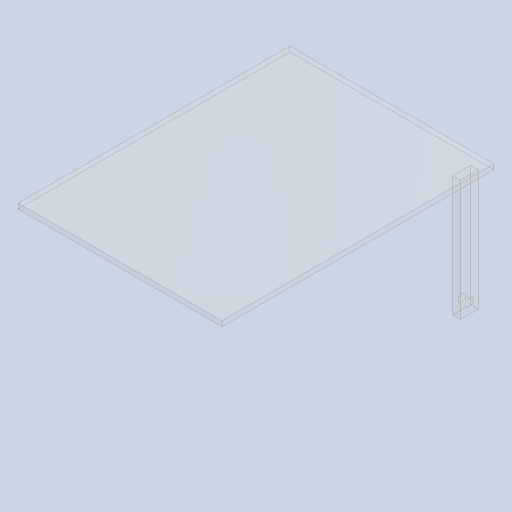
# Autodesk Inventor part: Enclosure Lid
Saved by Autodesk Inventor 2024 (Build 280153000, 153)
## iProperties
Created: 2025-03-05
Part Number: Enclosure Lid
Material: Generic
Document SubType Name: Modeling
Designer: Kemper Room 121
Density: 1 g/cm^3
Appearance: Polycarbonate - Clear
Author: Kemper Room 121
Autodesk Inventor part; units mm, degrees
ref_plane "YZ Plane" through (0, 0, 0) normal (1, 0, 0) x (0, 1, 0)
ref_plane "XZ Plane" through (0, 0, 0) normal (0, 1, 0) x (-1, 0, 0)
ref_plane "XY Plane" through (0, 0, 0) normal (0, 0, 1) x (1, 0, 0)
sketch "Sketch1" plane through (0, 0, 0) normal (0, 1, 0) x (-1, 0, 0)
  line L0 (0, 0) -> (79.5, 0)
  line L1 (79.5, 0) -> (79.5, -106)
  line L2 (79.5, -106) -> (0, -106)
  line L3 (0, -106) -> (0, 0)
  dimension "d6" = 106
  dimension "d7" = 79.5
  constraints: 8 end point, 2 parallel, 1 horizontal, 1 perpendicular
  measures "d6" distance of L0.end L1.end
  measures "d7" distance of L0.start L0.end
extrude "Extrusion1" add sketch "Sketch1" along normal blind 2
sketch "Sketch2" plane through (0, 0, 0) normal (0, -1, 0) x (1, 0, 0)
  line L0 (0, -106) -> (-79.5, -106) projected
  line L1 (0, 0) -> (0, -106) projected
  line L2 (-79.5, 0) -> (0, 0) projected
  line L3 (-79.5, -106) -> (-79.5, 0) projected
  line L4 (-3, -103) -> (-6, -103)
  line L5 (-6, -103) -> (-6, -96)
  line L6 (-6, -96) -> (-3, -96)
  line L7 (-3, -96) -> (-3, -103)
  dimension "d10" = 7
  dimension "d11" = 3
  dimension "d12" = 3
  dimension "d13" = 3
  constraints: 8 end point, 2 parallel, 1 horizontal, 1 perpendicular
  measures "d10" distance of L6.end L4.start
  measures "d11" distance between parallel lines of L1 L7
  measures "d12" distance between parallel lines of L0 L4
  measures "d13" distance of L4.start L4.end
extrude "Extrusion2" add sketch "Sketch2" along normal blind 48 contours L4 L5 L6 L7
sketch "Sketch3" plane through (-3, 0, -96) normal (1, 0, 0) x (0, 0, -1)
  circle A0 centre (3.5, -43) radius 1.5
  line L0 (7, -48) -> (0, -48) projected
  line L1 (7, 0) -> (7, -48) projected
  point P0 (-96, 0)
  dimension "d14" = 5
  dimension "d16" = 3
  dimension "d22" = 3.5
  constraints: 1 centre point
  measures "d14" distance from line of L0 A0.centre
  measures "d16" diameter of A0
  measures "d22" distance from line of L1 A0.centre
extrude "Extrusion3" cut sketch "Sketch3" against normal blind 33
sketch "Sketch4" plane through (-3, 0, -96) normal (1, 0, 0) x (0, 0, -1)
  circle A0 centre (3.5, -43) radius 1.5 projected
  line L0 (0, 0) -> (7, 0) projected
  line L1 (0, 0) -> (0, -48) projected
  line L2 (7, -48) -> (0, -48) projected
  line L3 (7, 0) -> (7, -48) projected
  line L4 (0, -48) -> (7, -48)
  line L5 (7, -48) -> (7, -47)
  line L6 (7, -47) -> (0, -47)
  line L7 (0, -47) -> (0, -48)
  point P0 (-96, 0)
  point P1 (0, -47)
  dimension "d19" = 1
  constraints: 8 end point, 2 parallel, 1 horizontal, 1 perpendicular, 1 point on line
  measures "d19" distance between parallel lines of L2 L6
extrude "Extrusion4" cut sketch "Sketch4" against normal blind 33 contours L6 L3 L2 L1
body "Solid1"
